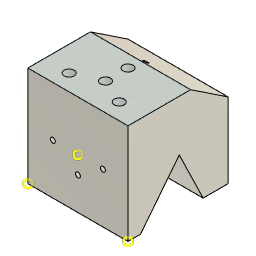
2024-03-20-Suètone-crab-03 (Autodesk Fusion 360 design; units mm, degrees)
Autodesk Fusion 360 part; units mm, degrees
sketch "Esquisse1" plane through (0, 0, 0) normal (0, 0, 1) x (1, 0, 0)
  line L0 (40, 40) -> (-40, 40)
  line L1 (-40, 40) -> (-40, -40)
  line L2 (-40, -40) -> (40, -40)
  line L3 (40, -40) -> (40, 40)
  line L4 (40, 40) -> (-40, -40) construction
  line L5 (-40, 40) -> (40, -40) construction
  dimension "d1" = 80
  dimension "d2" = 80
  constraint horizontal L0
  constraint perpendicular L0 L1
  constraint parallel L0 L2
  constraint parallel L1 L3
  constraint coincident L4 origin
  constraint coincident L5 origin
  measures "d1" distance of L1.end L2.end
  measures "d2" distance of L0.end L1.end
extrude "Extrusion1" add sketch "Esquisse1" along normal blind 80 makes body 1
sketch "Esquisse4" plane through (0, 0, 80) normal (0, 0, 1) x (-1, 0, 0)
  line L0 (-40, 40) -> (-40, -40)
  line L1 (-40, -40) -> (40, -40)
  line L2 (40, -40) -> (40, 40)
  line L3 (40, 40) -> (-40, 40)
  circle A0 centre (0, 18) radius 4
  circle A1 centre (0, 0) radius 4
  circle A2 centre (-20, 27) radius 4
  circle A3 centre (20, 27) radius 4
  dimension "d5" = 8
  dimension "d6" = 8
  dimension "d7" = 8
  dimension "d8" = 8
  constraint coincident A1.centre origin
  measures "d5" diameter of A0
  measures "d6" diameter of A1
  measures "d7" diameter of A2
  measures "d8" diameter of A3
extrude "Extrusion2" cut sketch "Esquisse4" against normal blind 95 contours A0 | A1 | A2 | A3 bodies 1
sketch "Esquisse6" plane through (-40, 0, 20) normal (-1, 0, 0) x (0, -1, 0)
sketch "Esquisse8" plane through (40, 0, 0) normal (1, 0, 0) x (0, 1, 0)
  line L0 (-40, 0) -> (40, 0)
  line L1 (40, 0) -> (40, 80)
  line L2 (40, 80) -> (-40, 80)
  line L3 (-40, 80) -> (-40, 0)
  line L4 (-30, 0) -> (0.95, 39.3693)
  line L5 (40, 0) -> (20, 0)
  line L6 (0.95, 39.3693) -> (20, 0)
  dimension "d12" = 20
  constraint coincident L0.end L1.start
  constraint perpendicular L1 L5
  measures "d12" distance of L0.end L5.end
sketch "Esquisse9" plane through (0, -40, 0) normal (0, -1, 0) x (1, 0, 0)
  point P0 (40, 0)
  point P1 (0, 40)
  point P2 (-40, 0)
extrude "Extrusion3" cut sketch "Esquisse8" against normal blind 175 contours L0 L4 L6 bodies 1
sketch "Esquisse10" plane through (40, 0, 0) normal (1, 0, 0) x (0, 1, 0)
  line L0 (0.95, 39.3693) -> (20, 0)
  line L1 (20, 0) -> (40, 0)
  line L2 (40, 0) -> (40, 80)
  line L3 (40, 80) -> (-40, 80)
  line L4 (-40, 80) -> (-40, 0)
  line L5 (-40, 0) -> (-30, 0)
  line L6 (-30, 0) -> (0.95, 39.3693)
  line L7 (10, 80) -> (40, 60)
ref_plane "Plan de construction1" through (40, 25, 70) normal (0, -0.5547, -0.83205) x (0, 0.83205, -0.5547)
split "Scinder1" by plane through (40, 25, 70) normal (0, -0.5547, -0.83205) bodies 1 makes body 2 at (-13.3333, -40, 26.6667)
delete_body "RemoveBody1" bodies 1
sketch "Esquisse11" plane through (0, 0, 80) normal (0, 0, 1) x (-1, 0, 0)
  line L0 (-40, -10) -> (40, -10)
  line L1 (40, -10) -> (40, 40)
  line L2 (40, 40) -> (-40, 40)
  line L3 (-40, 40) -> (-40, -10)
  circle A0 centre (-20, 27) radius 4
  circle A1 centre (0, 0) radius 4
  circle A2 centre (20, 27) radius 4
  circle A3 centre (0, 18) radius 4
sketch "Esquisse12" plane through (0, -40, 0) normal (0, -1, 0) x (1, 0, 0)
  line L0 (-40, 0) -> (40, 0)
  line L1 (40, 0) -> (40, 80)
  line L2 (40, 80) -> (-40, 80)
  line L3 (-40, 80) -> (-40, 0)
  line L4 (0, 80) -> (0, 0)
  constraint midpoint L2 L4.start
  constraint coincident L4.end origin
ref_plane "Plan de construction2" through (0, -40, 40) normal (1, 0, 0) x (0, 0, -1)
sketch "Esquisse15" plane through (0, -40, 0) normal (0, -1, 0) x (1, 0, 0)
  line L0 (-40, 0) -> (40, 0)
  line L1 (40, 0) -> (40, 80)
  line L2 (40, 80) -> (-40, 80)
  line L3 (-40, 80) -> (-40, 0)
  circle A0 centre (-20, 40) radius 2
  circle A1 centre (20, 40) radius 2
  circle A2 centre (0, 26) radius 2
  dimension "d21" = 4
  dimension "d22" = 4
  dimension "d23" = 4
  measures "d21" diameter of A0
  measures "d22" diameter of A1
  measures "d23" diameter of A2
extrude "Extrusion4" cut sketch "Esquisse15" against normal blind 10 contours A0 | A1 bodies 2
extrude "Extrusion5" cut sketch "Esquisse15" against normal blind 20 contours A2 bodies 2
sketch "Esquisse16" plane through (0, 40, 60) normal (0, 0.5547, 0.83205) x (-1, 0, 0)
  line L0 (40, 0) -> (40, 36.0555)
  line L1 (40, 36.0555) -> (-40, 36.0555)
  line L2 (-40, 36.0555) -> (-40, 0)
  line L3 (-40, 0) -> (40, 0)
  circle A0 centre (0, 31) radius 2
  dimension "d28" = 4
  measures "d28" diameter of A0
extrude "Extrusion6" cut sketch "Esquisse16" against normal blind 20 contours A0 bodies 2
sketch "Esquisse17" plane through (0, 0, 0) normal (0, 0, -1) x (1, 0, 0)
  line L0 (-40, 30) -> (-22.6458, 30)
  arc A0 (-17.3542, 30) -> (-22.6458, 30) centre (-20, 27) ccw
  line L1 (-17.3542, 30) -> (17.3542, 30)
  arc A1 (22.6458, 30) -> (17.3542, 30) centre (20, 27) ccw
  line L2 (22.6458, 30) -> (40, 30)
  line L3 (40, 30) -> (40, 40)
  line L4 (40, 40) -> (-40, 40)
  line L5 (-40, 40) -> (-40, 30)
  line L6 (37, 37) -> (-37, 37)
  line L7 (-37, 37) -> (-37, 33)
  line L8 (-37, 33) -> (37, 33)
  line L9 (37, 33) -> (37, 37)
  line L10 (37, 37) -> (-37, 33) construction
  line L11 (-37, 37) -> (37, 33) construction
  line L12 (37, -33) -> (-37, -33)
  line L13 (-37, -33) -> (-37, -37)
  line L14 (-37, -37) -> (37, -37)
  line L15 (37, -37) -> (37, -33)
  line L16 (37, -33) -> (-37, -37) construction
  line L17 (-37, -33) -> (37, -37) construction
  point P0 (0, 35)
  point P1 (0, -35)
  dimension "d31" = 74
  dimension "d32" = 4
  dimension "d33" = 74
  dimension "d34" = 4
  constraint horizontal L6
  constraint perpendicular L6 L7
  constraint parallel L6 L8
  constraint parallel L7 L9
  constraint coincident L10 P0
  constraint coincident L11 P0
  constraint horizontal L12
  constraint perpendicular L12 L13
  constraint parallel L12 L14
  constraint parallel L13 L15
  constraint coincident L16 P1
  constraint coincident L17 P1
  measures "d31" distance of L7.end L8.end
  measures "d32" distance of L6.end L7.end
  measures "d33" distance of L13.end L14.end
  measures "d34" distance of L12.end L13.end
extrude "Extrusion7" add sketch "Esquisse17" along normal blind 3 contours L6 L7 L8 L9 | L12 L13 L14 L15 bodies 2
sketch "Esquisse18" plane through (0, 0, 80) normal (0, 0, 1) x (-1, 0, 0)
